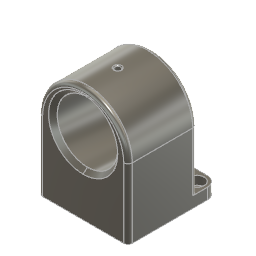
BASE_ASM (Autodesk Fusion 360 archive; units mm, degrees)
design "MIC_MOUNT"
Autodesk Fusion 360 part; units mm, degrees
sketch "Sketch1" plane through (0, 0, 0) normal (0, 1, 0) x (1, 0, 0)
  line L0 (-26, -6) -> (26, -6)
  line L1 (26, -6) -> (26, 6)
  line L2 (26, 6) -> (-26, 6)
  line L3 (-26, 6) -> (-26, -6)
  line L4 (-26, -6) -> (26, 6) construction
  line L5 (26, -6) -> (-26, 6) construction
  line L6 (20, 0) -> (-20, 0) construction
  point P0 (-20, 0)
  point P1 (20, 0)
  dimension "d1" = 52
  dimension "d2" = 12
  dimension "d4" = 20
  dimension "d5" = 20
  constraint horizontal L0
  constraint perpendicular L0 L1
  constraint parallel L0 L2
  constraint parallel L1 L3
  constraint coincident L4 origin
  constraint coincident L5 origin
  constraint coincident P1 L6.start
  constraint coincident P0 L6.end
  constraint horizontal L6
  measures "d1" distance of L1.end L2.end
  measures "d2" distance of L0.end L1.end
  measures "d4" distance of origin P0
  measures "d5" distance of origin P1
extrude "Extrude1" add sketch "Sketch1" against normal blind 6.5
hole "Hole1" at (-20, 0, 0) at (20, 0, 0) direction (0, -1, 0) diameter 5 end through all counterbore diameter 8.5 counterbore depth 5
sketch "Sketch2" plane through (0, 0, 6) normal (0, 0, 1) x (1, 0, 0)
  line L0 (26, 0) -> (-26, 0)
  line L1 (-26, 0) -> (-26, -6.5)
  line L2 (-26, -6.5) -> (26, -6.5)
  line L3 (26, -6.5) -> (26, 0)
  line L4 (-26, -6.5) -> (26, -6.5)
  line L5 (26, -6.5) -> (26, 60)
  line L6 (26, 60) -> (-26, 60)
  line L7 (-26, 60) -> (-26, -6.5)
  dimension "d12" = 52
  dimension "d13" = 26
  dimension "d19" = 60
  constraint horizontal L4
  constraint vertical L5
  constraint horizontal L6
  constraint vertical L7
  constraint coincident L1.end L4
  measures "d12" distance of L5.end L6.end
  measures "d13" distance of origin L7
  measures "d19" distance of origin L6
extrude "Extrude2" add sketch "Sketch2" along normal blind 40
ref_plane "WorkPlane1" through (0, 60, 46) normal (0, 0.087156, 0.996195) x (-1, 0, 0)
sketch "Sketch3" plane through (0, 4.4497, 50.86) normal (0, 0.087156, 0.996195) x (-1, 0, 0)
  circle A0 centre (0, -32.5) radius 17.5
  line L0 (0, 0) -> (0, -38.5685) construction
  dimension "d17" = 35
  dimension "d22" = 32.5
  constraint coincident L0.start origin
  constraint vertical L0
  constraint coincident A0.centre L0
  measures "d17" diameter of A0
  measures "d22" distance of L0.start A0.centre
extrude "Extrude3" cut sketch "Sketch3" against normal through all
fillet "Fillet1" radius 26 2 edges at (-26, 60, 26) (26, 60, 26)
fillet "Fillet2" radius 2.5 6 edges at (26, 17, 6) (0, 60, 6) (-26, 17, 6) (-26, 13.75, 46) (0, 60, 46) (26, 13.75, 46)
chamfer "Chamfer2" distance 2.5 angle 45 2 edges at (0, 15.5822, 6) (0, 19.0818, 46)
fillet "Fillet3" radius 6 2 edges at (26, -3.25, -6) (-26, -3.25, -6)
ref_plane "WorkPlane3" through (0, 60, 29.2895) normal (0, 1, 0) x (1, 0, 0)
sketch "Sketch5" plane through (0, 60, 0) normal (0, 1, 0) x (1, 0, 0)
  line L0 (-23.5, -6) -> (23.5, -6)
  point P0 (0, -26)
  dimension "d35" = 20
  measures "d35" distance of P0 L0
hole "Hole3" at (0, 60, 26) direction (0, -1, 0) diameter 3.5 depth 20 tip angle 180
chamfer "Chamfer3" distance 0.5 angle 45 2 edges at (1.75, 59.941, 26) (-1.75, 59.941, 26)

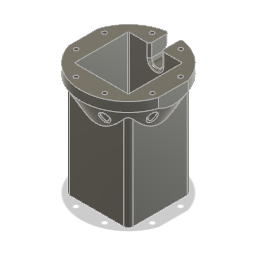
design "MOTOR_MOUNT"
Autodesk Fusion 360 part; units mm, degrees
sketch "Sketch2" plane through (0, 0, 0) normal (0, 1, 0) x (1, 0, 0)
  circle A0 centre (0, 0) radius 50
  dimension "d3" = 100
  constraint coincident A0.centre origin
  measures "d3" diameter of A0
extrude "Extrude1" add sketch "Sketch2" along normal blind 10
sketch "Sketch3" plane through (0, 0, 0) normal (0, -1, 0) x (1, 0, 0)
  circle A0 centre (0, 0) radius 50
  line L0 (-28.5, -28.5) -> (28.5, -28.5)
  line L1 (28.5, -28.5) -> (28.5, 28.5)
  line L2 (28.5, 28.5) -> (-28.5, 28.5)
  line L3 (-28.5, 28.5) -> (-28.5, -28.5)
  line L4 (-28.5, -28.5) -> (28.5, 28.5) construction
  line L5 (28.5, -28.5) -> (-28.5, 28.5) construction
  dimension "d6" = 57
  dimension "d7" = 57
  constraint horizontal L0
  constraint perpendicular L0 L1
  constraint parallel L0 L2
  constraint parallel L1 L3
  constraint coincident L4 A0.centre
  constraint coincident L5 A0.centre
  constraint coincident A0.centre origin
  measures "d6" distance of L0.end L1.end
  measures "d7" distance of L1.end L2.end
extrude "Extrude2" cut sketch "Sketch3" against normal up to surface (10 mm away) contours L0 L1 L2 L3
sketch "Sketch4" plane through (0, 0, 0) normal (0, -1, 0) x (1, 0, 0)
  line L0 (-28.5, 28.5) -> (28.5, 28.5)
  line L1 (28.5, 28.5) -> (28.5, -28.5)
  line L2 (28.5, -28.5) -> (-28.5, -28.5)
  line L3 (-28.5, -28.5) -> (-28.5, 28.5)
  circle A0 centre (0, 0) radius 50
  line L4 (-33.5, -33.5) -> (33.5, -33.5)
  line L5 (33.5, -33.5) -> (33.5, 33.5)
  line L6 (33.5, 33.5) -> (-33.5, 33.5)
  line L7 (-33.5, 33.5) -> (-33.5, -33.5)
  line L8 (-33.5, -33.5) -> (33.5, 33.5) construction
  line L9 (33.5, -33.5) -> (-33.5, 33.5) construction
  dimension "d10" = 67
  dimension "d11" = 67
  constraint horizontal L4
  constraint perpendicular L4 L5
  constraint parallel L4 L6
  constraint parallel L5 L7
  constraint coincident L8 A0.centre
  constraint coincident L9 A0.centre
  constraint coincident A0.centre origin
  measures "d10" distance of L5.end L6.end
  measures "d11" distance of L4.end L5.end
extrude "Extrude3" add sketch "Sketch4" along normal blind 73.5 contours L4 L5 L6 L7
sketch "Sketch5" plane through (0, -73.5, 0) normal (0, -1, 0) x (1, 0, 0)
  line L0 (28.5, -28.5) -> (-28.5, -28.5)
  line L1 (-28.5, -28.5) -> (-28.5, 28.5)
  line L2 (-28.5, 28.5) -> (28.5, 28.5)
  line L3 (28.5, 28.5) -> (28.5, -28.5)
  line L4 (-33.5, 33.5) -> (-33.5, -33.5)
  line L5 (-33.5, -33.5) -> (33.5, -33.5)
  line L6 (33.5, -33.5) -> (33.5, 33.5)
  line L7 (33.5, 33.5) -> (-33.5, 33.5)
  circle A0 centre (0, 0) radius 33.5
  circle A1 centre (0, 0) radius 28.25
  dimension "d14" = 56.5
  constraint coincident A0.centre A1.centre
  constraint tangent L4 A0
  measures "d14" diameter of A1
extrude "Extrude4" add sketch "Sketch5" along normal blind 35 contours L0 A0 | L0 L1 L2 L3 A0 | L3 A0 | L1 A0 | L2 A0
sketch "Sketch6" plane through (0, -73.5, 0) normal (0, -1, 0) x (1, 0, 0)
  arc A0 (-33.5, 0) -> (-28.5, -17.6068) centre (0, 0) ccw
  line L0 (-33.5, 0) -> (-33.5, -33.5)
  line L1 (-33.5, -33.5) -> (0, -33.5)
  arc A1 (-17.6068, -28.5) -> (0, -33.5) centre (0, 0) ccw
  line L2 (-17.6068, -28.5) -> (-28.5, -28.5)
  line L3 (-28.5, -28.5) -> (-28.5, -17.6068)
  circle A2 centre (0, 0) radius 33.5
  line L4 (-33.5, -33.5) -> (33.5, -33.5)
  line L5 (33.5, -33.5) -> (33.5, 33.5)
  line L6 (33.5, 33.5) -> (-33.5, 33.5)
  line L7 (-33.5, 33.5) -> (-33.5, -33.5)
  line L8 (-33.5, -33.5) -> (33.5, 33.5) construction
  line L9 (33.5, -33.5) -> (-33.5, 33.5) construction
  constraint horizontal L4
  constraint perpendicular L4 L5
  constraint parallel L4 L6
  constraint parallel L5 L7
  constraint coincident L8 A0.centre
  constraint coincident L9 A0.centre
  constraint coincident L0.end L1.start
  constraint coincident A0.centre A1.centre
extrude "Extrude5" add sketch "Sketch6" along normal up to surface (35 mm away) contours A0 L0 L1 A1 L2 L3 A2 L4 L7 | A2 L6 L7 | L2 L3 A2 | A2 L5 L6 | A2 L4 L5
sketch "Sketch7" plane through (0, -73.5, 0) normal (0, 1, 0) x (-1, 0, 0)
  circle A0 centre (0, 0) radius 28.25
  line L0 (28.5, -28.5) -> (28.5, 28.5)
  line L1 (28.5, 28.5) -> (-28.5, 28.5)
  line L2 (-28.5, 28.5) -> (-28.5, -28.5)
  line L3 (-28.5, -28.5) -> (28.5, -28.5)
  line L4 (-23.5, 23.5) -> (23.5, 23.5)
  line L5 (23.5, 23.5) -> (23.5, -23.5)
  line L6 (23.5, -23.5) -> (-23.5, -23.5)
  line L7 (-23.5, -23.5) -> (-23.5, 23.5)
  line L8 (-23.5, 23.5) -> (23.5, -23.5) construction
  line L9 (23.5, 23.5) -> (-23.5, -23.5) construction
  point P0 (23.5, 23.5)
  point P1 (23.5, -23.5)
  point P2 (-23.5, -23.5)
  point P3 (-23.5, 23.5)
  dimension "d20" = 47
  dimension "d21" = 47
  constraint horizontal L4
  constraint perpendicular L4 L5
  constraint parallel L4 L6
  constraint parallel L5 L7
  constraint coincident L8 A0.centre
  constraint coincident L9 A0.centre
  constraint coincident A0.centre origin
  constraint coincident P0 L4.end
  constraint coincident P1 L5.end
  constraint coincident P2 L6.end
  constraint coincident P3 L4.start
  measures "d20" distance of P1 P2
  measures "d21" distance of P3 P2
hole "Hole1" at (-23.5, -73.5, -23.5) at (23.5, -73.5, -23.5) at (23.5, -73.5, 23.5) at (-23.5, -73.5, 23.5) direction (0, -1, 0) diameter 3.5 depth 25 tip angle 180
fillet "Fillet1" radius 1 4 edges at (-22.8672, -73.5, -25.1316) (-22.8672, -73.5, 21.8684) (24.1328, -73.5, 21.8684) (24.1328, -73.5, -25.1316)
chamfer "Chamfer1" distance 1 angle 45 1 edges at (-26.3382, -73.5, 10.2156)
fillet "Fillet2" radius 5 4 edges at (-33.5, -54.25, -33.5) (33.5, -54.25, -33.5) (33.5, -54.25, 33.5) (-33.5, -54.25, 33.5)
sketch "Sketch8" plane through (0, 0, 0) normal (1, 0, 0) x (0, 0, -1)
  line L0 (50, 10) -> (-50, 10)
  line L1 (50, 0) -> (-50, 0)
  line L2 (-50, 0) -> (-32.6607, -30.0326)
  line L3 (-32.6607, -30.0326) -> (-32.6607, 0)
  dimension "d30" = 60
  constraint coincident L1.end L2.start
  constraint coincident L1 L3.end
  constraint perpendicular L1 L3
  measures "d30" angle of L1 L2
revolve "Revolve1" add sketch "Sketch8" angle 360 about axis through (0, 1.75, 0) along (0, 1, 0)
extrude "Extrude6" cut 4 faces at (-23.768, 0, 25.8793) (25.8793, 0, 23.768) (-23.768, 0, -25.8793) (25.8793, 0, -23.768) along direction (0, 1, 0) up to surface end surface through (-28.5, -30.0326, -15.9521) normal (0, 1, 0) offset 0
ref_plane "WorkPlane1" through (0, -30, 0) normal (0, 1, 0) x (1, 0, 0)
sketch "Sketch10" plane through (0, -30, 0) normal (0, 1, 0) x (1, 0, 0)
  point P0 (-40, -15)
  point P1 (-40.2953, 15)
  dimension "d37" = 40
  dimension "d38" = 30
  dimension "d39" = 15
  measures "d37" horizontal distance of origin P0
  measures "d38" vertical distance of P0 P1
  measures "d39" vertical distance of origin P0
hole "Hole2" at (-40.2953, -30, -15) at (-40, -30, 15) direction (0, 1, 0) diameter 4.25 depth 50 tip angle 180 counterbore diameter 7.25 counterbore depth 35
chamfer "Chamfer2" distance 1 angle 45 2 edges at (-38.7774, -12.2514, 18.4123) (-41.609, -11.7754, -11.6217)
pattern_circular "C-Pattern1" count 4 over 360 about axis through (0, 1.75, 0) along (0, 1, 0) of "Hole2", "Chamfer2"
sketch "Sketch11" plane through (0, 0, 0) normal (0, 1, 0) x (1, 0, 0)
  line L0 (-47.5, 54.4271) -> (47.5, 54.4271)
  line L1 (47.5, 54.4271) -> (47.5, -54.4271)
  line L2 (47.5, -54.4271) -> (-47.5, -54.4271)
  line L3 (-47.5, -54.4271) -> (-47.5, 54.4271)
  line L4 (-47.5, 54.4271) -> (47.5, -54.4271) construction
  line L5 (47.5, 54.4271) -> (-47.5, -54.4271) construction
  line L6 (56.2445, -64.4468) -> (-56.2445, -64.4468)
  line L7 (-56.2445, -64.4468) -> (-56.2445, 64.4468)
  line L8 (-56.2445, 64.4468) -> (56.2445, 64.4468)
  line L9 (56.2445, 64.4468) -> (56.2445, -64.4468)
  line L10 (56.2445, -64.4468) -> (-56.2445, 64.4468) construction
  line L11 (-56.2445, -64.4468) -> (56.2445, 64.4468) construction
  dimension "d48" = 95
  constraint horizontal L0
  constraint perpendicular L0 L1
  constraint parallel L0 L2
  constraint parallel L1 L3
  constraint coincident L4 origin
  constraint coincident L5 origin
  constraint horizontal L6
  constraint perpendicular L6 L7
  constraint parallel L6 L8
  constraint parallel L7 L9
  constraint coincident L10 origin
  constraint coincident L11 origin
  measures "d48" distance of L1.end L2.end
extrude "Extrude7" cut sketch "Sketch11" along normal through all and the other way through all
sketch "Sketch12" plane through (0, 10, 0) normal (0, 1, 0) x (-1, 0, 0)
  line L0 (-28.5, 28.5) -> (28.5, 28.5)
  line L1 (28.5, 28.5) -> (28.5, -28.5)
  line L2 (28.5, -28.5) -> (-28.5, -28.5)
  line L3 (-28.5, -28.5) -> (-28.5, 28.5)
  circle A0 centre (40, 15) radius 2.125
  circle A1 centre (40.2953, -15) radius 2.125
  circle A2 centre (-15, 40) radius 2.125
  circle A3 centre (15, 40.2953) radius 2.125
  circle A4 centre (-40, -15) radius 2.125
  circle A5 centre (-40.2953, 15) radius 2.125
  circle A6 centre (15, -40) radius 2.125
  circle A7 centre (-15, -40.2953) radius 2.125
  line L4 (47.5, -15.6125) -> (47.5, 15.6125)
  arc A8 (47.5, 15.6125) -> (-47.5, 15.6125) centre (0, 0) ccw
  line L5 (-47.5, 15.6125) -> (-47.5, -15.6125)
  arc A9 (-47.5, -15.6125) -> (47.5, -15.6125) centre (0, 0) ccw
  line L6 (6.25, -25) -> (-6.25, -25)
  line L7 (-6.25, -25) -> (-6.25, -55)
  line L8 (-6.25, -55) -> (6.25, -55)
  line L9 (6.25, -55) -> (6.25, -25)
  line L10 (6.25, -25) -> (-6.25, -55) construction
  line L11 (-6.25, -25) -> (6.25, -55) construction
  point P0 (0, -40)
  dimension "d51" = 12.5
  dimension "d52" = 30
  dimension "d53" = 40
  constraint horizontal L6
  constraint perpendicular L6 L7
  constraint parallel L6 L8
  constraint parallel L7 L9
  constraint coincident L10 P0
  constraint coincident L11 P0
  measures "d51" distance of L7.end L8.end
  measures "d52" distance of L6.end L7.end
  measures "d53" distance of A8.centre P0
extrude "Extrude8" cut sketch "Sketch12" against normal blind 20 contours L2 L6 L7 L9 | L2 A9 L7 L9 | A9 L7 L8 L9
fillet "Fillet4" radius 6.25 2 edges at (-6.25, -10, -36.1413) (6.25, -10, -36.1413)
fillet "Fillet5" radius 2.5 9 edges at (6.25, -1.8965, -48.504) (4.5572, -8.026, -45.1367) (-4.5572, -8.026, -45.1367) (-6.25, -1.8965, -48.504) (-6.25, 5, -49.6078) (-6.25, 3.125, -28.5) (0, -10, -28.5) (6.25, 3.125, -28.5) (6.25, 5, -49.6078)
fillet "Fillet6" radius 1 4 edges at (28.5, -31.75, -28.5) (28.5, -31.75, 28.5) (-28.5, -31.75, 28.5) (-28.5, -31.75, -28.5)
equation "d10 = 57.000 mm + 10 mm"
equation "d11 = 57.000 mm + 10 mm"
equation "d57 = ( 12.5 / 2 ) * 1 mm"

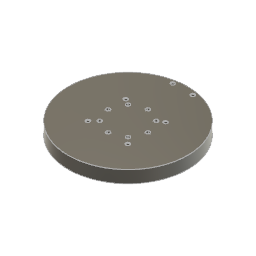
design "MONITOR_MOUNT"
Autodesk Fusion 360 part; units mm, degrees
sketch "Sketch1" plane through (0, 0, 0) normal (0, 1, 0) x (1, 0, 0)
  circle A0 centre (0, 0) radius 120
  dimension "d1" = 240
  constraint coincident A0.centre origin
  measures "d1" diameter of A0
extrude "Extrude1" add sketch "Sketch1" along normal blind 25
sketch "Sketch2" plane through (0, 0, 0) normal (0, -1, 0) x (1, 0, 0)
  circle A0 centre (0, 0) radius 120
  circle A1 centre (0, 0) radius 25.25
  dimension "d4" = 50.5
  constraint coincident A0.centre A1.centre
  measures "d4" diameter of A1
extrude "Extrude2" cut sketch "Sketch2" against normal blind 21 contours A1
sketch "Sketch8" plane through (0, 0, 0) normal (0, -1, 0) x (1, 0, 0)
  circle A0 centre (0, 0) radius 25.25
  circle A1 centre (0, 0) radius 120
  circle A2 centre (0, 0) radius 47.75
  dimension "d51" = 95.5
  constraint coincident A0.centre A1.centre
  measures "d51" diameter of A2
extrude "Extrude5" cut sketch "Sketch8" against normal blind 5.5 contours A2
sketch "Sketch9" plane through (0, 5.5, 0) normal (0, -1, 0) x (1, 0, 0)
  circle A0 centre (0, 0) radius 25.25
  circle A1 centre (0, 0) radius 47.75
  point P0 (0, 40)
  dimension "d54" = 40
  measures "d54" distance of A0.centre P0
hole "Hole5" at (0, 5.5, 40) direction (0, 1, 0) diameter 4 end through all
chamfer "Chamfer8" distance 0.5 angle 45 1 edges at (0.7232, 5.5, 41.8647)
sketch "Sketch10" plane through (0, 25, 0) normal (0, 1, 0) x (-1, 0, 0)
  circle A0 centre (0, 40) radius 2
  circle A1 centre (0, 0) radius 120
  line L0 (-3.625, 37.9071) -> (0, 35.8142)
  line L1 (0, 35.8142) -> (3.625, 37.9071)
  line L2 (3.625, 37.9071) -> (3.625, 42.0929)
  line L3 (3.625, 42.0929) -> (0, 44.1858)
  line L4 (0, 44.1858) -> (-3.625, 42.0929)
  line L5 (-3.625, 42.0929) -> (-3.625, 37.9071)
  point P0 (0, 40)
  dimension "d58" = 7.25
  constraint coincident P0 A0.centre
  measures "d58" distance of L2 L5
extrude "Extrude6" cut sketch "Sketch10" against normal blind 10 contours A0 | L0 L1 L2 L3 L4 L5
pattern_circular "C-Pattern3" count 8 over 360 about axis through (0, 1.75, 0) along (0, 1, 0) of "Hole5", "Chamfer8", "Extrude6"
ref_plane "WorkPlane1" through (0, 0, 140) normal (0, 0, 1) x (1, 0, 0)
sketch "Sketch3" plane through (0, 0, 140) normal (0, 0, 1) x (1, 0, 0)
  line L0 (120, 25) -> (-120, 25)
  circle A0 centre (0, 10) radius 5
  point P0 (0, 10)
  dimension "d8" = 15
  dimension "d14" = 10
  constraint coincident P0 A0.centre
  measures "d8" distance of P0 L0
  measures "d14" diameter of A0
hole "Hole1" [suppressed]
extrude "Extrude3" [suppressed]
chamfer "Chamfer1" [suppressed]
chamfer "Chamfer2" [suppressed]
pattern_circular "C-Pattern1" [suppressed]
ref_plane "WorkPlane2" through (0, 12.125, 0) normal (0.707107, 0, 0.707107) x (0, 1, 0)
ref_plane "WorkPlane3" through (98.9949, 12.125, 98.9949) normal (0.707107, 0, 0.707107) x (0, 1, 0)
sketch "Sketch5" plane through (98.9949, 0, 98.9949) normal (0.707107, 0, 0.707107) x (0, 1, 0)
  line L0 (25, -120) -> (25, 120)
  circle A0 centre (10, 0) radius 5
  point P0 (10, 0)
  dimension "d23" = 15
  dimension "d24" = 10
  constraint coincident P0 A0.centre
  measures "d23" distance of P0 L0
  measures "d24" diameter of A0
hole "Hole2" [suppressed]
extrude "Extrude4" [suppressed]
chamfer "Chamfer4" [suppressed]
pattern_circular "C-Pattern2" [suppressed]
sketch "Sketch6" plane through (0, 25, 0) normal (0, 1, 0) x (-1, 0, 0)
  circle A0 centre (0, 0) radius 120
  line L0 (-40, -35.5) -> (40, -35.5) construction
  line L1 (40, -35.5) -> (40, 40.5) construction
  line L2 (40, 40.5) -> (-40, 40.5) construction
  line L3 (-40, 40.5) -> (-40, -35.5) construction
  line L4 (-40, -35.5) -> (40, 40.5) construction
  line L5 (40, -35.5) -> (-40, 40.5) construction
  line L6 (0, -69.3411) -> (0, 34.1101) construction
  point P0 (0, 2.5)
  point P1 (-40, 40.5)
  point P2 (40, 40.5)
  point P3 (40, -35.5)
  point P4 (-40, -35.5)
  dimension "d36" = 80
  dimension "d37" = 76
  dimension "d82" = 2.5
  constraint horizontal L0
  constraint perpendicular L0 L1
  constraint parallel L0 L2
  constraint parallel L1 L3
  constraint coincident L4 P0
  constraint coincident L5 P0
  constraint coincident P1 L2.end
  constraint coincident P2 L1.end
  constraint coincident L0.end L1.start
  constraint coincident P4 L0.start
  constraint perpendicular L0 L6
  constraint coincident P0 L6
  constraint coincident A0.centre L6
  measures "d36" distance of P2 P1
  measures "d37" distance of P4 P1
  measures "d82" distance of A0.centre P0
hole "Hole3" at (40, 25, 40.5) at (-40, 25, 40.5) at (-40, 25, -35.5) at (40, 25, -35.5) direction (0, -1, 0) diameter 6 depth 7.5 tip angle 180
chamfer "Chamfer5" distance 1 angle 45 4 edges at (41.0848, 25, 37.703) (41.0848, 25, -38.297) (-38.9152, 25, -38.297) (-38.9152, 25, 37.703)
sketch "Sketch7" plane through (0, 25, 0) normal (0, 1, 0) x (-1, 0, 0)
  circle A0 centre (0, 0) radius 120
  line L0 (-110, 92.5) -> (110, 92.5)
  line L1 (110, 92.5) -> (110, -92.5)
  line L2 (110, -92.5) -> (-110, -92.5)
  line L3 (-110, -92.5) -> (-110, 92.5)
  line L4 (-110, 92.5) -> (110, -92.5) construction
  line L5 (110, 92.5) -> (-110, -92.5) construction
  line L6 (32.3274, -27.2009) -> (31.2441, -31.2441)
  line L7 (31.2441, -31.2441) -> (27.2009, -32.3274)
  line L8 (3.625, -42.0929) -> (0, -44.1858)
  line L9 (0, -44.1858) -> (-3.625, -42.0929)
  line L10 (-27.2009, -32.3274) -> (-31.2441, -31.2441)
  line L11 (-31.2441, -31.2441) -> (-32.3274, -27.2009)
  line L12 (-42.0929, -3.625) -> (-44.1858, 0)
  line L13 (-44.1858, 0) -> (-42.0929, 3.625)
  line L14 (-32.3274, 27.2009) -> (-31.2441, 31.2441)
  line L15 (-31.2441, 31.2441) -> (-27.2009, 32.3274)
  line L16 (-3.625, 42.0929) -> (0, 44.1858)
  line L17 (0, 44.1858) -> (3.625, 42.0929)
  line L18 (27.2009, 32.3274) -> (31.2441, 31.2441)
  line L19 (31.2441, 31.2441) -> (32.3274, 27.2009)
  line L20 (42.0929, 3.625) -> (44.1858, 0)
  line L21 (44.1858, 0) -> (42.0929, -3.625)
  circle A1 centre (40, -35.5) radius 4
  circle A2 centre (-40, 40.5) radius 4
  line L22 (25.3245, 25.3245) -> (24.2411, 29.3676)
  line L23 (24.2411, 29.3676) -> (27.2009, 32.3274)
  line L24 (32.3274, 27.2009) -> (29.3676, 24.2411)
  line L25 (29.3676, 24.2411) -> (25.3245, 25.3245)
  line L26 (35.8142, 0) -> (37.9071, 3.625)
  line L27 (37.9071, 3.625) -> (42.0929, 3.625)
  line L28 (42.0929, -3.625) -> (37.9071, -3.625)
  line L29 (37.9071, -3.625) -> (35.8142, 0)
  line L30 (25.3245, -25.3245) -> (29.3676, -24.2411)
  line L31 (29.3676, -24.2411) -> (32.3274, -27.2009)
  line L32 (27.2009, -32.3274) -> (24.2411, -29.3676)
  line L33 (24.2411, -29.3676) -> (25.3245, -25.3245)
  line L34 (0, -35.8142) -> (3.625, -37.9071)
  line L35 (3.625, -37.9071) -> (3.625, -42.0929)
  line L36 (-3.625, -42.0929) -> (-3.625, -37.9071)
  line L37 (-3.625, -37.9071) -> (0, -35.8142)
  line L38 (-25.3245, -25.3245) -> (-24.2411, -29.3676)
  line L39 (-24.2411, -29.3676) -> (-27.2009, -32.3274)
  line L40 (-32.3274, -27.2009) -> (-29.3676, -24.2411)
  line L41 (-29.3676, -24.2411) -> (-25.3245, -25.3245)
  line L42 (-35.8142, 0) -> (-37.9071, -3.625)
  line L43 (-37.9071, -3.625) -> (-42.0929, -3.625)
  line L44 (-42.0929, 3.625) -> (-37.9071, 3.625)
  line L45 (-37.9071, 3.625) -> (-35.8142, 0)
  line L46 (-25.3245, 25.3245) -> (-29.3676, 24.2411)
  line L47 (-29.3676, 24.2411) -> (-32.3274, 27.2009)
  line L48 (-27.2009, 32.3274) -> (-24.2411, 29.3676)
  line L49 (-24.2411, 29.3676) -> (-25.3245, 25.3245)
  line L50 (0, 35.8142) -> (-3.625, 37.9071)
  line L51 (-3.625, 37.9071) -> (-3.625, 42.0929)
  line L52 (3.625, 42.0929) -> (3.625, 37.9071)
  line L53 (3.625, 37.9071) -> (0, 35.8142)
  circle A3 centre (-40, -35.5) radius 4
  circle A4 centre (40, 40.5) radius 4
  point P0 (-20, -110)
  point P1 (20, -110)
  dimension "d42" = 20
  dimension "d43" = 110
  dimension "d44" = 20
  dimension "d45" = 110
  dimension "d46" = 220
  dimension "d47" = 185
  constraint horizontal L0
  constraint perpendicular L0 L1
  constraint parallel L0 L2
  constraint parallel L1 L3
  constraint coincident L4 A0.centre
  constraint coincident L5 A0.centre
  constraint coincident A0.centre origin
  measures "d42" horizontal distance of A0.centre P1
  measures "d43" vertical distance of A0.centre P1
  measures "d44" horizontal distance of A0.centre P0
  measures "d45" vertical distance of A0.centre P0
  measures "d46" distance of L1.end L2.end
  measures "d47" distance of L0.end L1.end
hole "Hole4" at (-20, 25, -110) at (20, 25, -110) direction (0, -1, 0) diameter 6 end through all
chamfer "Chamfer7" distance 1 angle 45 2 edges at (-18.9152, 25, -112.797) (21.0848, 25, -112.797)
sketch "Sketch12" plane through (0, 0, 0) normal (0, -1, 0) x (1, 0, 0)
  circle A0 centre (0, 0) radius 120
  line L0 (0, 0) -> (-65.1468, 112.8375)
  line L1 (0, 0) -> (63.7699, 110.4528)
  line L2 (0, 0) -> (0, 154.4828) construction
  circle A1 centre (0, 0) radius 62.5
  circle A2 centre (0, 0) radius 105
  circle A3 centre (0, 0) radius 47.75
  circle A4 centre (-20, -110) radius 3
  circle A5 centre (20, -110) radius 3
  dimension "d65" = 30
  dimension "d66" = 30
  dimension "d67" = 125
  dimension "d68" = 210
  constraint coincident A0.centre L0.start
  constraint vertical L2
  measures "d65" angle of L1 L2
  measures "d66" angle of L0 L2
  measures "d67" diameter of A1
  measures "d68" diameter of A2
extrude "Extrude7" cut sketch "Sketch12" against normal blind 15 contours L0 L1 A1 A2 picked at (40.7036, 80.9337)
fillet "Fillet1" radius 5 4 edges at (52.5, 7.5, 90.9327) (-52.5, 7.5, 90.9327) (-31.25, 7.5, 54.1266) (31.25, 7.5, 54.1266)
pattern_circular "C-Pattern4" count 3 over 180 about axis through (0, 1.75, 0) along (0, 1, 0) both ways of "Extrude7", "Fillet1"
sketch "Sketch13" plane through (0, 0, 0) normal (0, -1, 0) x (1, 0, 0)
  circle A0 centre (0, 0) radius 120
  line L0 (0, 0) -> (71.9145, -102.7046)
  line L1 (0, 0) -> (-82.4086, -117.6916)
  line L2 (0, 0) -> (0, -83.8814) construction
  circle A1 centre (0, 0) radius 62.5
  circle A2 centre (0, 0) radius 90
  circle A3 centre (0, 0) radius 47.75
  line L3 (86.4942, -49.9375) -> (58.2961, -33.6573)
  arc A4 (56.2927, -27.1548) -> (58.2961, -33.6573) centre (60.7961, -29.3272) ccw
  arc A5 (56.2927, -27.1548) -> (56.2927, 27.1548) centre (0, 0) ccw
  arc A6 (58.2961, 33.6573) -> (56.2927, 27.1548) centre (60.7961, 29.3272) ccw
  line L4 (58.2961, 33.6573) -> (86.4942, 49.9375)
  arc A7 (93.4439, 47.8877) -> (86.4942, 49.9375) centre (88.9942, 45.6073) ccw
  arc A8 (93.4439, -47.8877) -> (93.4439, 47.8877) centre (0, 0) ccw
  arc A9 (86.4942, -49.9375) -> (93.4439, -47.8877) centre (88.9942, -45.6073) ccw
  line L5 (-86.4942, 49.9375) -> (-58.2961, 33.6573)
  arc A10 (-56.2927, 27.1548) -> (-58.2961, 33.6573) centre (-60.7961, 29.3272) ccw
  arc A11 (-56.2927, 27.1548) -> (-56.2927, -27.1548) centre (0, 0) ccw
  arc A12 (-58.2961, -33.6573) -> (-56.2927, -27.1548) centre (-60.7961, -29.3272) ccw
  line L6 (-58.2961, -33.6573) -> (-86.4942, -49.9375)
  arc A13 (-93.4439, -47.8877) -> (-86.4942, -49.9375) centre (-88.9942, -45.6073) ccw
  arc A14 (-93.4439, 47.8877) -> (-93.4439, -47.8877) centre (0, 0) ccw
  arc A15 (-86.4942, 49.9375) -> (-93.4439, 47.8877) centre (-88.9942, 45.6073) ccw
  line L7 (49.9375, 86.4942) -> (33.6573, 58.2961)
  arc A16 (27.1548, 56.2927) -> (33.6573, 58.2961) centre (29.3272, 60.7961) ccw
  arc A17 (27.1548, 56.2927) -> (-27.1548, 56.2927) centre (0, 0) ccw
  arc A18 (-33.6573, 58.2961) -> (-27.1548, 56.2927) centre (-29.3272, 60.7961) ccw
  line L8 (-33.6573, 58.2961) -> (-49.9375, 86.4942)
  arc A19 (-47.8877, 93.4439) -> (-49.9375, 86.4942) centre (-45.6073, 88.9942) ccw
  arc A20 (47.8877, 93.4439) -> (-47.8877, 93.4439) centre (0, 0) ccw
  arc A21 (49.9375, 86.4942) -> (47.8877, 93.4439) centre (45.6073, 88.9942) ccw
  circle A22 centre (-20, -110) radius 3
  circle A23 centre (20, -110) radius 3
  dimension "d75" = 35
  dimension "d76" = 35
  dimension "d77" = 180
  constraint coincident A0.centre L0.start
  constraint vertical L2
  measures "d75" angle of L1 L2
  measures "d76" angle of L0 L2
  measures "d77" diameter of A2
extrude "Extrude8" cut sketch "Sketch13" against normal up to surface (15 mm away) contours L0 L1 A1 A2
fillet "Fillet2" radius 5 4 edges at (-51.6219, 7.5, -73.7237) (-35.8485, 7.5, -51.197) (51.6219, 7.5, -73.7237) (35.8485, 7.5, -51.197)
chamfer "Chamfer9" distance 0.5 angle 45 2 edges at (18.9152, 0, -112.797) (-21.0848, 0, -112.797)
sketch "Sketch15" plane through (0, 25, 0) normal (0, 1, 0) x (-1, 0, 0)
  circle A0 centre (20, -110) radius 4
  circle A1 centre (40, -35.5) radius 4
  circle A2 centre (-40, 40.5) radius 4
  line L0 (25.3245, 25.3245) -> (24.2411, 29.3676)
  line L1 (24.2411, 29.3676) -> (27.2009, 32.3274)
  line L2 (27.2009, 32.3274) -> (31.2441, 31.2441)
  line L3 (31.2441, 31.2441) -> (32.3274, 27.2009)
  line L4 (32.3274, 27.2009) -> (29.3676, 24.2411)
  line L5 (29.3676, 24.2411) -> (25.3245, 25.3245)
  line L6 (35.8142, 0) -> (37.9071, 3.625)
  line L7 (37.9071, 3.625) -> (42.0929, 3.625)
  line L8 (42.0929, 3.625) -> (44.1858, 0)
  line L9 (44.1858, 0) -> (42.0929, -3.625)
  line L10 (42.0929, -3.625) -> (37.9071, -3.625)
  line L11 (37.9071, -3.625) -> (35.8142, 0)
  line L12 (25.3245, -25.3245) -> (29.3676, -24.2411)
  line L13 (29.3676, -24.2411) -> (32.3274, -27.2009)
  line L14 (32.3274, -27.2009) -> (31.2441, -31.2441)
  line L15 (31.2441, -31.2441) -> (27.2009, -32.3274)
  line L16 (27.2009, -32.3274) -> (24.2411, -29.3676)
  line L17 (24.2411, -29.3676) -> (25.3245, -25.3245)
  line L18 (0, -35.8142) -> (3.625, -37.9071)
  line L19 (3.625, -37.9071) -> (3.625, -42.0929)
  line L20 (3.625, -42.0929) -> (0, -44.1858)
  line L21 (0, -44.1858) -> (-3.625, -42.0929)
  line L22 (-3.625, -42.0929) -> (-3.625, -37.9071)
  line L23 (-3.625, -37.9071) -> (0, -35.8142)
  line L24 (-25.3245, -25.3245) -> (-24.2411, -29.3676)
  line L25 (-24.2411, -29.3676) -> (-27.2009, -32.3274)
  line L26 (-27.2009, -32.3274) -> (-31.2441, -31.2441)
  line L27 (-31.2441, -31.2441) -> (-32.3274, -27.2009)
  line L28 (-32.3274, -27.2009) -> (-29.3676, -24.2411)
  line L29 (-29.3676, -24.2411) -> (-25.3245, -25.3245)
  line L30 (-35.8142, 0) -> (-37.9071, -3.625)
  line L31 (-37.9071, -3.625) -> (-42.0929, -3.625)
  line L32 (-42.0929, -3.625) -> (-44.1858, 0)
  line L33 (-44.1858, 0) -> (-42.0929, 3.625)
  line L34 (-42.0929, 3.625) -> (-37.9071, 3.625)
  line L35 (-37.9071, 3.625) -> (-35.8142, 0)
  line L36 (-25.3245, 25.3245) -> (-29.3676, 24.2411)
  line L37 (-29.3676, 24.2411) -> (-32.3274, 27.2009)
  line L38 (-32.3274, 27.2009) -> (-31.2441, 31.2441)
  line L39 (-31.2441, 31.2441) -> (-27.2009, 32.3274)
  line L40 (-27.2009, 32.3274) -> (-24.2411, 29.3676)
  line L41 (-24.2411, 29.3676) -> (-25.3245, 25.3245)
  line L42 (0, 35.8142) -> (-3.625, 37.9071)
  line L43 (-3.625, 37.9071) -> (-3.625, 42.0929)
  line L44 (-3.625, 42.0929) -> (0, 44.1858)
  line L45 (0, 44.1858) -> (3.625, 42.0929)
  line L46 (3.625, 42.0929) -> (3.625, 37.9071)
  line L47 (3.625, 37.9071) -> (0, 35.8142)
  circle A3 centre (0, 0) radius 120
  circle A4 centre (-40, -35.5) radius 4
  circle A5 centre (40, 40.5) radius 4
  circle A6 centre (-20, -110) radius 4
  line L48 (110, 97.5) -> (-110, 97.5)
  line L49 (-110, 97.5) -> (-110, -92.5)
  line L50 (-110, -92.5) -> (110, -92.5)
  line L51 (110, -92.5) -> (110, 97.5)
  line L52 (110, 97.5) -> (-110, -92.5) construction
  line L53 (-110, 97.5) -> (110, -92.5) construction
  line L54 (40, -35.5) -> (-40, 40.5)
  line L55 (-40, -35.5) -> (40, 40.5)
  point P0 (0, 2.5)
  dimension "d86" = 220
  dimension "d87" = 190
  constraint horizontal L48
  constraint perpendicular L48 L49
  constraint parallel L48 L50
  constraint parallel L49 L51
  constraint coincident L52 P0
  constraint coincident L53 P0
  constraint coincident A1.centre L54.start
  constraint coincident A2.centre L54.end
  constraint coincident A4.centre L55.start
  constraint coincident A5.centre L55.end
  constraint midpoint P0 L54
  measures "d86" distance of L49.end L50.end
  measures "d87" distance of L48.end L49.end
ref_plane "WorkPlane4" through (0, 0, -121) normal (0, 0, 1) x (1, 0, 0)
sketch "Sketch16" plane through (0, 0, -121) normal (0, 0, 1) x (1, 0, 0)
  point P0 (0, 12.5)
  dimension "d89" = 12.5
  measures "d89" distance of origin P0
hole "Hole6" at (0, 12.5, -121) direction (0, 0, 1) diameter 6 depth 15 tip angle 180
chamfer "Chamfer10" distance 1 angle 45 1 edges at (-3, 12.5, -119.9625)
equation "d8 = 11 mm + 4 mm"

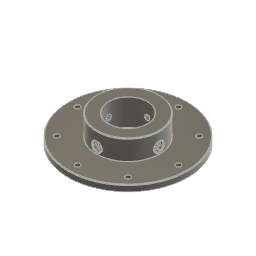
design "STEPPER_MOTOR_HUB"
Autodesk Fusion 360 part; units mm, degrees
sketch "Sketch1" plane through (0, 0, 0) normal (0, 1, 0) x (1, 0, 0)
  circle A0 centre (0, 0) radius 15.45
  circle A1 centre (0, 0) radius 25
  dimension "d1" = 50
  dimension "d2" = 30.9
  constraint coincident A0.centre A1.centre
  measures "d1" diameter of A1
  measures "d2" diameter of A0
extrude "Extrude1" add sketch "Sketch1" along normal blind 21
ref_plane "WorkPlane1" through (26, 0, 0) normal (1, 0, 0) x (0, 1, 0)
sketch "Sketch2" plane through (26, 0, 0) normal (1, 0, 0) x (0, 0, -1)
  point P0 (0, 10)
  dimension "d6" = 10
  measures "d6" distance of origin P0
hole "Hole1" at (26, 10, 0) direction (-1, 0, 0) diameter 4 depth 12 tip angle 180 counterbore diameter 7.25 counterbore depth 4
chamfer "Chamfer1" distance 0.5 angle 45 1 edges at (24.7358, 10, -3.625)
pattern_circular "C-Pattern1" count 4 over 360 about axis through (0, 1.75, 0) along (0, 1, 0) of "Hole1", "Chamfer1"
sketch "Sketch3" plane through (0, 0, 0) normal (0, -1, 0) x (1, 0, 0)
  circle A0 centre (0, 0) radius 15.45
  circle A1 centre (0, 0) radius 25
  circle A2 centre (0, 0) radius 47.5
  dimension "d15" = 95
  constraint coincident A0.centre A1.centre
  measures "d15" diameter of A2
extrude "Extrude2" add sketch "Sketch3" against normal blind 5 contours A2
chamfer "Chamfer2" distance 0.5 angle 45 1 edges at (-23.3082, 21, 9.0404)
sketch "Sketch4" plane through (0, 0, 0) normal (0, -1, 0) x (1, 0, 0)
  circle A0 centre (0, 0) radius 47.5
  circle A1 centre (0, 0) radius 15.45
  point P0 (0, 40)
  dimension "d19" = 40
  measures "d19" distance of A0.centre P0
hole "Hole2" at (0, 0, 40) direction (0, 1, 0) diameter 4 end through all counterbore diameter 7.25 counterbore depth 2
chamfer "Chamfer3" distance 0.5 angle 45 1 edges at (1.3109, 0, 43.3797)
pattern_circular "C-Pattern2" count 8 over 360 about axis through (0, 1.75, 0) along (0, 1, 0) of "Hole2", "Chamfer3"
chamfer "Chamfer4" distance 0.5 angle 45 1 edges at (-44.2855, 5, 17.1767)

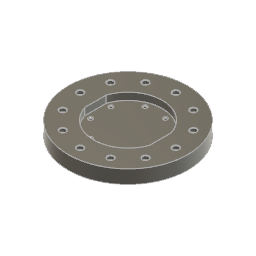
design "BASE_PIECE"
Autodesk Fusion 360 part; units mm, degrees
sketch "Sketch1" plane through (0, 0, 0) normal (0, 1, 0) x (1, 0, 0)
  circle A0 centre (0, 0) radius 87.5
  dimension "d1" = 175
  constraint coincident A0.centre origin
  measures "d1" diameter of A0
extrude "Extrude1" add sketch "Sketch1" along normal blind 20
sketch "Sketch2" plane through (0, 20, 0) normal (0, 1, 0) x (-1, 0, 0)
  circle A0 centre (0, 0) radius 87.5
  circle A1 centre (0, 0) radius 50.25
  line L0 (47.75, 86.5797) -> (-47.75, 86.5797)
  line L1 (-47.75, 86.5797) -> (-47.75, -86.5797)
  line L2 (-47.75, -86.5797) -> (47.75, -86.5797)
  line L3 (47.75, -86.5797) -> (47.75, 86.5797)
  line L4 (47.75, 86.5797) -> (-47.75, -86.5797) construction
  line L5 (-47.75, 86.5797) -> (47.75, -86.5797) construction
  dimension "d4" = 100.5
  dimension "d7" = 95.5
  constraint coincident A0.centre A1.centre
  constraint horizontal L0
  constraint perpendicular L0 L1
  constraint parallel L0 L2
  constraint parallel L1 L3
  constraint coincident L4 A0.centre
  constraint coincident L5 A0.centre
  measures "d4" diameter of A1
  measures "d7" distance of L1 L3
extrude "Extrude2" cut sketch "Sketch2" against normal blind 10.5 contours A1 L1 L3
sketch "Sketch4" plane through (0, 20, 0) normal (0, 1, 0) x (-1, 0, 0)
  line L0 (47.75, 15.6525) -> (47.75, -15.6525)
  arc A0 (-47.75, -15.6525) -> (47.75, -15.6525) centre (0, 0) ccw
  line L1 (-47.75, -15.6525) -> (-47.75, 15.6525)
  arc A1 (47.75, 15.6525) -> (-47.75, 15.6525) centre (0, 0) ccw
  circle A2 centre (0, 0) radius 87.5
  point P0 (15, -40)
  point P1 (-15, -40)
  dimension "d8" = 30
  dimension "d9" = 15
  dimension "d10" = 40
  dimension "d11" = 40
  measures "d8" horizontal distance of P0 P1
  measures "d9" horizontal distance of A0.centre P1
  measures "d10" vertical distance of A0.centre P1
  measures "d11" vertical distance of A0.centre P0
hole "Hole1" at (15, 20, -40) at (-15, 20, -40) direction (0, -1, 0) diameter 4.25 end through all
chamfer "Chamfer1" distance 1 angle 45 2 edges at (-14.2316, 9.5, -41.9812) (15.7684, 9.5, -41.9812)
sketch "Sketch5" plane through (0, 0, 0) normal (0, -1, 0) x (1, 0, 0)
  circle A0 centre (15, -40) radius 2.125
  circle A1 centre (-15, -40) radius 2.125
  circle A2 centre (0, 0) radius 87.5
  line L0 (-18.575, -42.064) -> (-15, -44.1281)
  line L1 (-15, -44.1281) -> (-11.425, -42.064)
  line L2 (-11.425, -42.064) -> (-11.425, -37.936)
  line L3 (-11.425, -37.936) -> (-15, -35.8719)
  line L4 (-15, -35.8719) -> (-18.575, -37.936)
  line L5 (-18.575, -37.936) -> (-18.575, -42.064)
  line L6 (11.425, -42.064) -> (15, -44.1281)
  line L7 (15, -44.1281) -> (18.575, -42.064)
  line L8 (18.575, -42.064) -> (18.575, -37.936)
  line L9 (18.575, -37.936) -> (15, -35.8719)
  line L10 (15, -35.8719) -> (11.425, -37.936)
  line L11 (11.425, -37.936) -> (11.425, -42.064)
  point P0 (-15, -40)
  point P1 (15, -40)
  dimension "d15" = 7.15
  dimension "d16" = 7.15
  constraint coincident P0 A1.centre
  constraint coincident A0.centre P1
  measures "d15" distance of L8 L11
  measures "d16" distance of L2 L5
extrude "Extrude3" cut sketch "Sketch5" against normal blind 5 contours A0 | A1 | L0 L1 L2 L3 L4 L5 | L6 L7 L8 L9 L10 L11
pattern_circular "C-Pattern1" count 4 over 360 about axis through (0, 1.75, 0) along (0, 1, 0) of "Hole1", "Chamfer1", "Extrude3"
sketch "Sketch6" plane through (0, 20, 0) normal (0, 1, 0) x (-1, 0, 0)
  line L0 (47.75, 15.6525) -> (47.75, -15.6525)
  arc A0 (-47.75, -15.6525) -> (47.75, -15.6525) centre (0, 0) ccw
  line L1 (-47.75, -15.6525) -> (-47.75, 15.6525)
  arc A1 (47.75, 15.6525) -> (-47.75, 15.6525) centre (0, 0) ccw
  circle A2 centre (0, 0) radius 87.5
  point P0 (0, -70)
  dimension "d21" = 70
  measures "d21" distance of A0.centre P0
hole "Hole2" at (0, 20, -70) direction (0, -1, 0) diameter 5.5 end through all counterbore diameter 8.75 counterbore depth 5.5
chamfer "Chamfer2" distance 0.5 angle 45 1 edges at (1.5821, 20, -74.0789)
pattern_circular "C-Pattern2" count 12 over 360 about axis through (0, 1.75, 0) along (0, 1, 0) of "Hole2", "Chamfer2"
